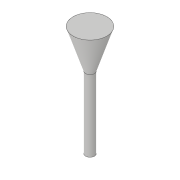
# Autodesk Inventor part: pour2
Saved by Autodesk Inventor 2018 (Build 220112000, 112)
## iProperties
Created: 2020-02-14
Part Number: pour2
Material: Generic
Document SubType Name: Modeling
Designer: Matt
Density: 1 g/cm^3
Appearance: Default
Author: Matt
Autodesk Inventor part; units mm, degrees
ref_plane "YZ Plane" through (0, 0, 0) normal (1, 0, 0) x (0, 1, 0)
ref_plane "XZ Plane" through (0, 0, 0) normal (0, 1, 0) x (-1, 0, 0)
ref_plane "XY Plane" through (0, 0, 0) normal (0, 0, 1) x (1, 0, 0)
sketch "Sketch1" plane through (0, 0, 0) normal (0, 0, 1) x (1, 0, 0)
  line L0 (0, 0) -> (3.175, 0)
  line L1 (3.175, 0) -> (3.175, 50.8553)
  line L2 (3.175, 50.8553) -> (11.9774, 78.3642)
  line L3 (11.9774, 78.3642) -> (0, 78.3642)
  line L4 (0, 78.3642) -> (0, 0)
  dimension "d0" = 3.175
  constraints: 10 end point, 2 perpendicular, 1 horizontal, 1 parallel
  measures "d0" distance of L0.start L0.end
revolve "Revolution1" add sketch "Sketch1" angle 360 about axis through (0, 78.3642, 0) along (0, -1, 0)
body "Solid1"
